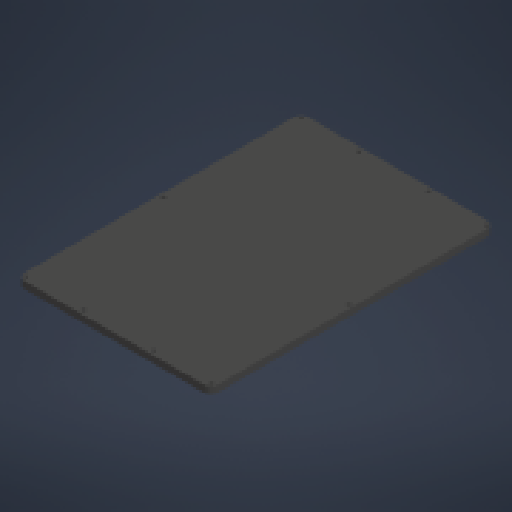
# Autodesk Inventor part: screen_case
Saved by Autodesk Inventor 2026.2 (Build 302298000, 298)
## iProperties
Created: 2026-01-27
Part Number: screen_case
Material: Generic
Document SubType Name: Modeling
Designer: test
Density: 1 g/cm^3
Appearance: Default
Author: test
Autodesk Inventor part; units mm, degrees
ref_plane "YZ Plane" through (0, 0, 0) normal (1, 0, 0) x (0, 1, 0)
ref_plane "XZ Plane" through (0, 0, 0) normal (0, 1, 0) x (-1, 0, 0)
ref_plane "XY Plane" through (0, 0, 0) normal (0, 0, 1) x (1, 0, 0)
sketch "Sketch1" plane through (0, 0, 0) normal (0, 1, 0) x (-1, 0, 0)
  line L0 (0, 0) -> (187, 0)
  line L1 (187, 0) -> (187, -274.11)
  line L2 (187, -274.11) -> (0, -274.11)
  line L3 (0, -274.11) -> (0, 0)
  dimension "d0" = 187
  dimension "d1" = 274.11
  constraints: 8 end point, 2 parallel, 1 horizontal, 1 perpendicular
  measures "d0" distance of L1.end L2.end
  measures "d1" distance of L0.end L1.end
extrude "Extrusion1" add sketch "Sketch1" along normal blind 6.6
fillet "Fillet1" radius 7 4 edges at (0, 3.3, 0) (-187, 3.3, 0) (-187, 3.3, -274.11) (0, 3.3, -274.11)
sketch "Sketch2" plane through (0, 0, 0) normal (0, -1, 0) x (1, 0, 0)
  line L0 (-9.5, -10.055) -> (-177.5, -10.055)
  line L1 (-177.5, -10.055) -> (-177.5, -264.055)
  line L2 (-177.5, -264.055) -> (-9.5, -264.055)
  line L3 (-9.5, -264.055) -> (-9.5, -10.055)
  arc A0 (-7, -274.11) -> (0, -267.11) centre (-7, -267.11) ccw projected
  line L4 (0, -7) -> (0, -267.11) projected
  arc A1 (0, -7) -> (-7, 0) centre (-7, -7) ccw projected
  line L5 (-180, 0) -> (-7, 0) projected
  arc A2 (-180, 0) -> (-187, -7) centre (-180, -7) ccw projected
  line L6 (-187, -267.11) -> (-187, -7) projected
  arc A3 (-187, -267.11) -> (-180, -274.11) centre (-180, -267.11) ccw projected
  line L7 (-7, -274.11) -> (-180, -274.11) projected
  line L8 (-7, -7) -> (-180, -267.11) construction
  line L9 (-177.5, -10.055) -> (-9.5, -264.055) construction
  point P0 (0, 0)
  point P1 (-93.5, -137.055)
  dimension "d5" = 254
  dimension "d6" = 168
  constraints: 12 end point, 2 midpoint, 2 parallel, 1 horizontal, 1 perpendicular
  measures "d5" distance of L2.end L0.start
  measures "d6" distance of L0.start L0.end
extrude "Extrusion2" add sketch "Sketch2" along normal blind 2 contours L3 L2 L1 L0
fillet "Fillet2" radius 7 4 edges at (-9.5, -1, -264.055) (-177.5, -1, -264.055) (-177.5, -1, -10.055) (-9.5, -1, -10.055)
sketch "Sketch3" plane through (0, 6.6, 0) normal (0, 1, 0) x (1, 0, 0)
  line L0 (0, 7) -> (0, 267.11) projected
  line L1 (0, 137.055) -> (-187, 137.055) construction
  line L2 (-187, 267.11) -> (-187, 7) projected
  line L3 (-7, 274.11) -> (-180, 274.11) projected
  line L4 (-93.5, 274.11) -> (-93.5, 0) construction
  line L5 (-180, 0) -> (-7, 0) projected
  circle A0 centre (-4, 137.055) radius 2
  circle A1 centre (-4, 4.5) radius 2
  circle A2 centre (-60, 4.5) radius 2
  circle A3 centre (-4, 269.61) radius 2
  line L6 (-4, 269.61) -> (-183, 269.61) construction
  line L7 (-183, 269.61) -> (-183, 4.5) construction
  line L8 (-183, 4.5) -> (-4, 4.5) construction
  line L9 (-4, 4.5) -> (-4, 269.61) construction
  circle A4 centre (-60, 269.61) radius 2
  circle A5 centre (-183, 137.055) radius 2
  circle A6 centre (-183, 4.5) radius 2
  circle A7 centre (-127, 4.5) radius 2
  circle A8 centre (-183, 269.61) radius 2
  circle A9 centre (-127, 269.61) radius 2
  point P0 (0, 0)
  dimension "d9" = 4
  dimension "d10" = 4
  dimension "d11" = 4
  dimension "d18" = 265.11
  dimension "d19" = 179
  dimension "d20" = 67
  constraints: 12 end point, 10 centre point, 7 symmetric about line, 5 midpoint, 2 coincident, 2 parallel, 2 point on line, 1 horizontal, 1 perpendicular, 7 other
  measures "d9" diameter of A0
  measures "d10" diameter of A1
  measures "d11" diameter of A2
  measures "d18" distance between parallel lines of L6 L8
  measures "d19" distance between parallel lines of L7 L9
  measures "d20" distance of A9.centre A4.centre
extrude "Extrusion4" cut sketch "Sketch3" against normal up to surface (6.6 mm away)
body "Solid1"
